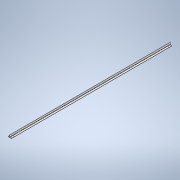
# Autodesk Inventor part: Lift.01.00.00.01
Saved by Autodesk Inventor 2021 (Build 250183000, 183)
## iProperties
Created: 2020-09-20
Part Number: Lift.01.00.00.01
Material: Типовые
Document SubType Name: Modeling
Designer: Kostya
Density: 1 g/cm^3
Appearance: По умолчанию
Author: Kostya
Autodesk Inventor part; units mm, degrees
ref_plane "YZ Plane" through (0, 0, 0) normal (1, 0, 0) x (0, 1, 0)
ref_plane "XZ Plane" through (0, 0, 0) normal (0, 1, 0) x (-1, 0, 0)
ref_plane "XY Plane" through (0, 0, 0) normal (0, 0, 1) x (1, 0, 0)
sketch "Эскиз1" plane through (0, 0, 0) normal (0, 0, 1) x (1, 0, 0)
  line L0 (0, 0) -> (0, 188.5182) construction
  line L1 (0, 0) -> (-63.5, 0)
  line L2 (-63.5, 0) -> (-63.5, 12.6983)
  line L3 (-63.5, 12.6983) -> (-8.7709, 15.8539)
  arc A0 (-8.7709, 15.8539) -> (-5.0012, 19.8473) centre (-9.0012, 19.8473) ccw
  line L4 (-5.0012, 19.8473) -> (-5.0012, 34.1273)
  arc A1 (-5.0012, 34.1273) -> (-8, 38) centre (-9.0012, 34.1273) ccw
  line L5 (-8, 38) -> (-8, 89)
  line L6 (-8, 89) -> (0, 89)
  line L7 (0, 0) -> (63.5, 0)
  line L8 (63.5, 0) -> (63.5, 12.6983)
  line L9 (63.5, 12.6983) -> (8.7709, 15.8539)
  arc A2 (5.0012, 19.8473) -> (8.7709, 15.8539) centre (9.0012, 19.8473) ccw
  line L10 (5.0012, 19.8473) -> (5.0012, 34.1273)
  arc A3 (8, 38) -> (5.0012, 34.1273) centre (9.0012, 34.1273) ccw
  line L11 (8, 38) -> (8, 89)
  line L12 (8, 89) -> (0, 89)
  dimension "d1" = 63.5
  dimension "d2" = 54.82
  dimension "d3" = 14.28
  dimension "d4" = 8
  dimension "d5" = 89
  dimension "d6" = 93.3
  dimension "d7" = 4
  dimension "d8" = 4
  dimension "d9" = 51
  constraints: 26 end point, 9 symmetric about line, 8 point on circle, 4 centre point, 3 tangent, 2 perpendicular, 2 vertical, 1 horizontal, 1 parallel, 1 point on line, 2 other
  measures "d1" distance between parallel lines of L2 L0
  measures "d2" distance of L2.end L3.end
  measures "d3" distance of L4.start L4.end
  measures "d4" distance between parallel lines of L0 L5
  measures "d5" distance between parallel lines of L1 L6
  measures "d6" angle of L2 L3
  measures "d7" radius of A0
  measures "d8" radius of A1
  measures "d9" distance of L5.start L5.end
extrude "Выдавливание1" add sketch "Эскиз1" along normal mid plane 6000
sketch "Эскиз3" plane through (-63.5, 0, 3000) normal (0, -1, 0) x (1, 0, 0)
  line L0 (127, -6000) -> (127, 0) projected
  line L1 (0, 0) -> (127, 0) projected
  line L2 (0, -6000) -> (0, 0) projected
  line L3 (127, -6000) -> (0, -6000) projected
  line L4 (55.5, -6000) -> (55.5, 0) projected
  line L5 (71.5, 0) -> (55.5, 0) projected
  line L6 (71.5, -6000) -> (71.5, 0) projected
  line L7 (55.5, -6000) -> (71.5, -6000) projected
  line L8 (127, 0) -> (72.2709, 0) projected
  line L9 (54.7291, 0) -> (0, 0) projected
  point P0 (63.5, -3000)
  point P1 (99.6355, -38.1)
  point P2 (99.6355, -114.3)
  point P3 (27.3645, -38.1)
  point P4 (27.3645, -114.3)
  point P5 (99.6355, 0)
  point P6 (27.3645, 0)
  dimension "d14" = 38.1
  dimension "d15" = 76.2
  constraints: 4 vertical alignment, 2 horizontal alignment, 2 midpoint
  measures "d14" distance from line of L1 point (27.365, -38.1)
  measures "d15" distance of point (27.365, -114.3) point (27.365, -38.1)
hole "Отверстие1" at (36.1355, 0, 2961.9) at (36.1355, 0, 2885.7) at (-36.1355, 0, 2961.9) at (-36.1355, 0, 2885.7) direction (0, 1, 0) diameter 17 end through all
sketch "Эскиз4" plane through (-63.5, 0, 3000) normal (0, -1, 0) x (1, 0, 0)
  circle A0 centre (27.3645, -38.1) radius 8.5 projected
  circle A1 centre (99.6355, -38.1) radius 8.5 projected
  circle A2 centre (99.6355, -114.3) radius 8.5 projected
  circle A3 centre (27.3645, -114.3) radius 8.5 projected
  line L0 (127, -6000) -> (127, 0) projected
  line L1 (0, 0) -> (127, 0) projected
  line L2 (0, -6000) -> (0, 0) projected
  line L3 (127, -6000) -> (0, -6000) projected
  line L4 (127, 0) -> (127, -6000) projected
  line L5 (127, -152.5) -> (0, -152.5)
  line L6 (0, -6000) -> (0, 0) projected
  point P0 (63.5, -3000)
  dimension "d23" = 152.5
  constraints: 2 end point, 2 point on line, 1 horizontal
  measures "d23" distance between parallel lines of L1 L5
extrude "Выдавливание2" cut sketch "Эскиз4" against normal blind 1 contours L5 L2 L1 L0
mirror "Зеркальное отражение2" about plane through (0, 0, 0) normal (0, 0, 1) of "Отверстие1", "Выдавливание2"
equation "\"d8\" = d7"
